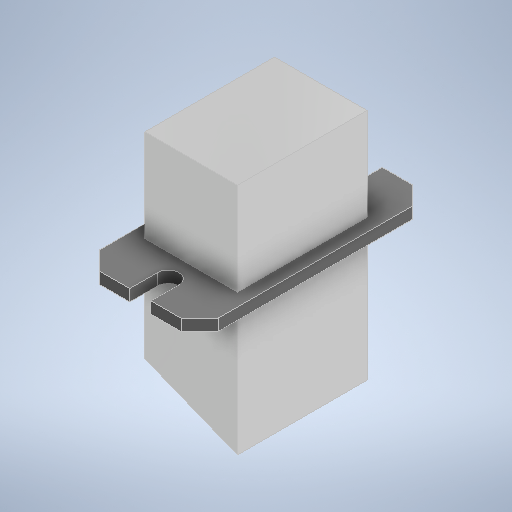
# Autodesk Inventor part: Molex 1061141150 Fiber-Optic Passthrough
Saved by Autodesk Inventor 2025 (Build 290162000, 162)
## iProperties
Created: 2025-06-10
Part Number: Molex 1061141150 Fiber-Optic Passthrough
Material: Generic
Document SubType Name: Modeling
Designer: Caleb Fangmeier
Density: 1 g/cm^3
Appearance: Gray
Author: Caleb Fangmeier
Autodesk Inventor part; units mm, degrees
ref_plane "YZ Plane" through (0, 0, 0) normal (1, 0, 0) x (0, 1, 0)
ref_plane "XZ Plane" through (0, 0, 0) normal (0, 1, 0) x (-1, 0, 0)
ref_plane "XY Plane" through (0, 0, 0) normal (0, 0, 1) x (1, 0, 0)
sketch "Sketch1" plane through (0, 0, 0) normal (0, 1, 0) x (-1, 0, 0)
  line L0 (-4.4, -12.5) -> (4.4, -12.5)
  line L1 (6.4, -10.5) -> (6.4, 10.5)
  line L2 (4.4, 12.5) -> (-4.4, 12.5)
  line L3 (-6.4, 10.5) -> (-6.4, -10.5)
  line L4 (-6.4, -12.5) -> (6.4, 12.5) construction
  line L5 (6.4, -12.5) -> (-6.4, 12.5) construction
  line L6 (6.4, 10.5) -> (4.4, 12.5)
  line L7 (-4.4, 12.5) -> (-6.4, 10.5)
  line L8 (6.4, -10.5) -> (4.4, -12.5)
  line L9 (-4.4, -12.5) -> (-6.4, -10.5)
  line L10 (0, 12.5) -> (0, 9.5) construction
  line L11 (-1.15, 12.5) -> (-1.15, 9.5)
  line L12 (1.15, 9.5) -> (1.15, 12.5)
  arc A0 (1.15, 12.5) -> (-1.15, 12.5) centre (0, 12.5) ccw
  arc A1 (-1.15, 9.5) -> (1.15, 9.5) centre (0, 9.5) ccw
  line L13 (0, -12.5) -> (0, -9.5) construction
  line L14 (1.15, -12.5) -> (1.15, -9.5)
  line L15 (-1.15, -9.5) -> (-1.15, -12.5)
  arc A2 (-1.15, -12.5) -> (1.15, -12.5) centre (0, -12.5) ccw
  arc A3 (1.15, -9.5) -> (-1.15, -9.5) centre (0, -9.5) ccw
  point P0 (0, 0)
  point P1 (0, 11)
  point P2 (0, -11)
  dimension "d0" = 25
  dimension "d1" = 12.8
  dimension "d2" = 2
  dimension "d3" = 2
  dimension "d4" = 2
  dimension "d5" = 2
  dimension "d6" = 2
  dimension "d7" = 2
  dimension "d8" = 2
  dimension "d9" = 2
  dimension "d10" = 2.3
  dimension "d11" = 2.3
  dimension "d12" = 3
  dimension "d13" = 3
  constraints: 36 end point, 9 point on line, 8 point on circle, 8 tangent, 6 midpoint, 4 centre point, 4 parallel, 2 perpendicular, 1 horizontal
  measures "d0" distance of L5.start L4.end
  measures "d1" distance of L4.end L5.end
  measures "d2" distance of L1.end L4.end
  measures "d3" distance of L2.start L4.end
  measures "d4" distance of L2.end L5.end
  measures "d5" distance of L3.start L5.end
  measures "d6" distance of L1.start L5.start
  measures "d7" distance of L0.end L5.start
  measures "d8" distance of L0.start L4.start
  measures "d9" distance of L3.end L4.start
  measures "d10" distance between parallel lines of L12 L11
  measures "d11" distance between parallel lines of L14 L15
  measures "d12" distance from line of L2 L10.end
  measures "d13" distance of L13.end L13.start
extrude "Extrusion1" add sketch "Sketch1" along normal blind 1.25 contours L9 L3 L7 L2 L11 A1 L12 L6 L1 L8 L0 L14 A3 L15
sketch "Sketch2" plane through (0, 1.25, 0) normal (0, 1, 0) x (1, 0, 0)
  line L0 (5, 7) -> (-5, 7)
  line L1 (-5, 7) -> (-5, -7)
  line L2 (-5, -7) -> (5, -7)
  line L3 (5, -7) -> (5, 7)
  line L4 (5, 7) -> (-5, -7) construction
  line L5 (-5, 7) -> (5, -7) construction
  point P0 (0, 0)
  dimension "d16" = 10
  dimension "d17" = 14
  constraints: 12 end point, 2 midpoint, 2 parallel, 1 horizontal, 1 perpendicular
  measures "d16" distance of L1.end L2.end
  measures "d17" distance of L0.end L1.end
extrude "Extrusion2" add sketch "Sketch2" along normal blind 10
sketch "Sketch3" plane through (0, 0, 0) normal (0, -1, 0) x (1, 0, 0)
  line L0 (5, 7) -> (-5, 7)
  line L1 (-5, 7) -> (-5, -7)
  line L2 (-5, -7) -> (5, -7)
  line L3 (5, -7) -> (5, 7)
  line L4 (5, 7) -> (-5, -7) construction
  line L5 (-5, 7) -> (5, -7) construction
  point P0 (0, 0)
  dimension "d20" = 10
  dimension "d21" = 14
  constraints: 12 end point, 2 midpoint, 2 parallel, 1 horizontal, 1 perpendicular
  measures "d20" distance of L1.end L2.end
  measures "d21" distance of L0.end L1.end
extrude "Extrusion3" add sketch "Sketch3" along normal blind 14
sketch "Sketch4" plane through (-5, 0, 7) normal (0, 0, 1) x (1, 0, 0)
  line L0 (10, 0) -> (10, -14) projected
  line L1 (10, -14) -> (0, -10)
  line L2 (0, 0) -> (0, -14) projected
  line L3 (10, -14) -> (0, -14) projected
  point P0 (5, 0)
  dimension "d24" = 4
  constraints: 2 end point, 1 point on line
  measures "d24" distance of L2.end L1.end
extrude "Extrusion4" cut sketch "Sketch4" against normal through all
equation "\"d3\" = d2"
equation "\"d4\" = d2"
equation "\"d5\" = d4"
equation "\"d6\" = d2"
equation "\"d7\" = d6"
equation "\"d8\" = d2"
equation "\"d9\" = d8"
equation "\"d11\" = d10"
equation "\"d13\" = d12"
body "Solid1"
